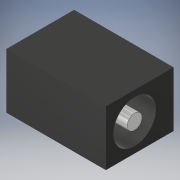
# Autodesk Inventor part: Barrel Jack small
Saved by Autodesk Inventor 2019 (Build 230136000, 136)
## iProperties
Created: 2020-02-13
Part Number: Barrel Jack small
Material: Generic
Document SubType Name: Modeling
Designer: close
Density: 1 g/cm^3
Appearance: Default
Author: close
Autodesk Inventor part; units mm, degrees
ref_plane "YZ Plane" through (0, 0, 0) normal (1, 0, 0) x (0, 1, 0)
ref_plane "XZ Plane" through (0, 0, 0) normal (0, 1, 0) x (-1, 0, 0)
ref_plane "XY Plane" through (0, 0, 0) normal (0, 0, 1) x (1, 0, 0)
sketch "Sketch1" plane through (0, 0, 0) normal (0, 1, 0) x (-1, 0, 0)
  line L0 (0, 0) -> (9, 0)
  line L1 (9, 0) -> (9, -6.12)
  line L2 (9, -6.12) -> (0, -6.12)
  line L3 (0, -6.12) -> (0, 0)
  dimension "d0" = 6.12
  dimension "d1" = 9
  constraints: 8 end point, 2 parallel, 1 horizontal, 1 perpendicular
  measures "d0" distance of L0.end L1.end
  measures "d1" distance of L1.end L2.end
extrude "Extrusion1" add sketch "Sketch1" along normal blind 5
sketch "Sketch2" plane through (0, 0, 0) normal (1, 0, 0) x (0, 0, -1)
  circle A0 centre (2.6, 2.5) radius 1.925
  circle A1 centre (2.6, 2.5) radius 0.675
  line L0 (6.12, 0) -> (0, 0) projected
  line L1 (0, 5) -> (6.12, 5) projected
  line L2 (0, 0) -> (0, 5) projected
  dimension "d4" = 3.85
  dimension "d5" = 1.35
  dimension "d6" = 5
  dimension "d7" = 2.5
  dimension "d8" = 2.6
  constraints: 2 centre point, 1 coincident
  measures "d4" diameter of A0
  measures "d5" diameter of A1
  measures "d6" distance between parallel lines of L0 L1
  measures "d7" distance from line of L1 A0.centre
  measures "d8" distance from line of L2 A0.centre
extrude "Extrusion2" cut sketch "Sketch2" against normal blind 7
equation "\"d7\" = 0.5 * d6"
body "Solid1"
